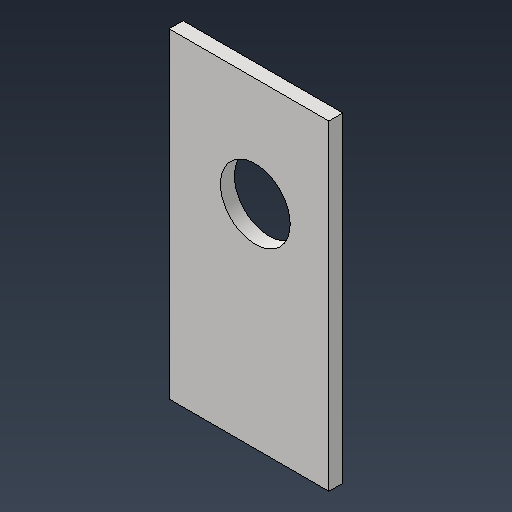
# Autodesk Inventor part: LeftGearboxCoverr
Saved by Autodesk Inventor 2026.2 (Build 302298010, 298A)
## iProperties
Created: 2026-04-13
Part Number: LeftGearboxCoverr
Material: Generic
Document SubType Name: Modeling
Designer: szymo
Density: 1 g/cm^3
Appearance: Default
Author: szymo
Autodesk Inventor part; units mm, degrees
ref_plane "YZ Plane" through (0, 0, 0) normal (1, 0, 0) x (0, 1, 0)
ref_plane "XZ Plane" through (0, 0, 0) normal (0, 1, 0) x (-1, 0, 0)
ref_plane "XY Plane" through (0, 0, 0) normal (0, 0, 1) x (1, 0, 0)
sketch "Sketch1" plane through (0, 0, 0) normal (0, 0, 1) x (1, 0, 0)
  circle A0 centre (14.7, -55.6371) radius 14.7 construction
  circle A1 centre (14.7, -55.6371) radius 14 construction
  circle A2 centre (14.7, -14.7) radius 14.7 construction
  circle A3 centre (14.7, -14.7) radius 14 construction
  line L0 (22.9, -65.6371) -> (0, -65.6371)
  line L1 (0, -65.6371) -> (0, -19.7)
  line L2 (0, -19.7) -> (22.9, -19.7)
  line L3 (22.9, -19.7) -> (22.9, -65.6371)
  circle A4 centre (12.35, -35.2722) radius 5 projected
  point P0 (0, 0)
  dimension "d0" = 6.5
  dimension "d4" = 4.7
  dimension "d7" = 19.7
  constraints: 8 end point, 2 parallel, 1 horizontal, 1 perpendicular, 1 tangent
  measures "d0" distance edge to line of A0 L3
  measures "d4" distance edge to line of A0 L0
extrude "Extrusion1" add sketch "Sketch1" against normal blind 2
body "Solid1"
